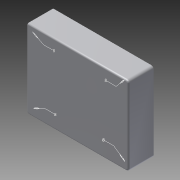
# Autodesk Inventor part: Boitier
Saved by Autodesk Inventor 2013 (Build 170138000, 138)
## iProperties
Created: 2013-04-17
Part Number: Boitier
Material: Plastique ABS
Document SubType Name: Modeling
Designer: dimercur
Density: 1.493 g/cm^3
Mass: 505.057 g
Surface Area: 353.982 cm^2
Volume: 338.283 cm^3
Author: dimercur
Autodesk Inventor part; units mm, degrees
ref_plane "YZ Plane" through (0, 0, 0) normal (1, 0, 0) x (0, 1, 0)
ref_plane "XZ Plane" through (0, 0, 0) normal (0, 1, 0) x (-1, 0, 0)
ref_plane "XY Plane" through (0, 0, 0) normal (0, 0, 1) x (1, 0, 0)
sketch "Esquisse1" plane through (0, 0, 0) normal (0, 1, 0) x (-1, 0, 0)
  line L0 (-46.9932, 34.5256) -> (73.6068, 34.5256)
  line L1 (73.6068, 34.5256) -> (73.6068, -58.9744)
  line L2 (73.6068, -58.9744) -> (-46.9932, -58.9744)
  line L3 (-46.9932, -58.9744) -> (-46.9932, 34.5256)
  point P0 (0, 0)
  dimension "d0" = 120.6
  dimension "d2" = 93.5
  constraints: 8 end point, 2 parallel, 1 horizontal, 1 perpendicular
  measures "d0" distance of L0.start L0.end
  measures "d2" distance of L2.end L0.start
extrude "Extrusion1" add sketch "Esquisse1" along normal blind 30
fillet "Congé1" radius 3 4 edges at (-73.6068, 15, -58.9744) (46.9932, 15, -58.9744) (-73.6068, 15, 34.5256) (46.9932, 15, 34.5256)
fillet "Congé2" radius 2 8 edges at (46.1146, 0, -58.0957) (46.9932, 0, -12.2244) (46.1146, 0, 33.647) (-13.3068, 0, 34.5256) (-72.7281, 0, 33.647) (-73.6068, 0, -12.2244) (-72.7281, 0, -58.0957) (-13.3068, 0, -58.9744)
shell "Coque1" thickness 2 removed faces 1 at (5.7932, 30, 3.359)
sketch "Esquisse2" plane through (-70.6068, 2, 32.5256) normal (0, 1, 0) x (1, 0, 0)
  line L0 (114.6, 0) -> (0, 0) projected
  arc A0 (114.6, 0) -> (115.6, 1) centre (114.6, 1) ccw projected
  line L1 (115.6, 88.5) -> (115.6, 1) projected
  arc A1 (115.6, 88.5) -> (114.6, 89.5) centre (114.6, 88.5) ccw projected
  line L2 (114.6, 89.5) -> (0, 89.5) projected
  arc A2 (0, 89.5) -> (-1, 88.5) centre (0, 88.5) ccw projected
  line L3 (-1, 1) -> (-1, 88.5) projected
  arc A3 (-1, 1) -> (0, 0) centre (0, 1) ccw projected
  circle A4 centre (7.1405, 82.078) radius 4
  circle A5 centre (108.4816, 82.078) radius 4
  circle A6 centre (108.4816, 4.0474) radius 4
  circle A7 centre (5.9552, 7.9983) radius 4
  point P0 (70.6068, 32.5256)
  dimension "d8" = 8
  dimension "d10" = 8
  dimension "d11" = 8
  dimension "d12" = 8
  constraints: 4 centre point
  measures "d8" diameter of A4
  measures "d10" diameter of A5
  measures "d11" diameter of A6
  measures "d12" diameter of A7
